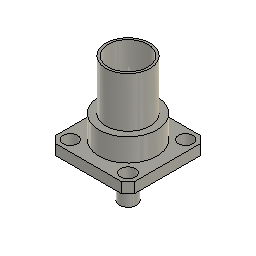
sBitx V3 radio aj6cu v1 (Autodesk Fusion 360 archive; units mm, degrees)
design "BNC connector"
Autodesk Fusion 360 part; units mm, degrees
sketch "Sketch1" plane through (0, 0, 0) normal (0, 1, 0) x (1, 0, 0) in component "BNC 4-hole panel mount"
  line L0 (-6.35, -9.3) -> (-8.75, -9.3)
  line L1 (-8.75, -9.3) -> (-8.75, -11.6)
  line L2 (-8.75, -11.6) -> (-6.35, -11.6)
  line L3 (-6.35, -11.6) -> (-6.35, -16.6)
  line L4 (-6.35, -16.6) -> (-4.85, -16.6)
  line L5 (-4.85, -16.6) -> (-4.85, -27.6)
  line L6 (0, -27.6) -> (0, 0)
  line L7 (-6.35, -9.3) -> (-6.35, -7.3)
  line L8 (-6.35, -7.3) -> (-1.9, -7.3)
  line L9 (-1.9, -7.3) -> (-1.9, 0)
  line L10 (0, 0) -> (-1.9, 0)
  line L11 (-4.85, -27.6) -> (-4.35, -27.6)
  line L12 (-4.35, -27.6) -> (-4.35, -14.6)
  line L13 (-4.35, -14.6) -> (-0.6, -14.6)
  line L14 (-0.6, -14.6) -> (-0.6, -24.1)
  line L15 (-0.6, -24.1) -> (0, -25.6)
  dimension "d3" = 1.9
  dimension "d4" = 2.3
  dimension "d5" = 5
  dimension "d6" = 8.75
  dimension "d9" = 4.85
  dimension "d10" = 6.35
  dimension "d11" = 2
  dimension "d21" = 0.5
  dimension "d22" = 0.6
  dimension "d23" = 1.5
  dimension "d24" = 13
  dimension "d25" = 27.6
  dimension "d26" = 11
  dimension "d27" = 16
  constraint perpendicular L0 L1
  constraint perpendicular L1 L2
  constraint perpendicular L2 L3
  constraint perpendicular L3 L4
  constraint perpendicular L4 L5
  constraint vertical L6
  constraint coincident L6.end L10.start
  constraint perpendicular L0 L7
  constraint perpendicular L7 L8
  constraint perpendicular L8 L9
  constraint perpendicular L9 L10
  constraint collinear L3 L7
  constraint perpendicular L5 L11
  constraint perpendicular L11 L12
  constraint perpendicular L12 L13
  constraint perpendicular L13 L14
  constraint coincident L6 L15.end
  measures "d3" distance of L6 L9
  measures "d4" distance of L0.end L1.end
  measures "d5" distance of L2 L4
  measures "d6" distance of L1 L6
  measures "d9" distance of L5 L6
  measures "d10" distance of L3 L6
  measures "d11" distance of L0 L8
  measures "d21" distance of L5 L12
  measures "d22" distance of L6 L14
  measures "d23" vertical distance of L14.end L15.end
  measures "d24" distance of L11.end L12.end
  measures "d25" vertical distance of L6.end L5.end
  measures "d26" distance of L13 L15.end
  measures "d27" distance of L2 L5.end
revolve "Revolve1" add sketch "Sketch1" angle 360 about axis through (0, 0, 27.6) along (0, 0, -1) in component "BNC 4-hole panel mount"
sketch "Sketch2" plane through (0, 0, 11.6) normal (0, 0, 1) x (-1, 0, 0) in component "BNC 4-hole panel mount"
  circle A0 centre (0, 0) radius 6.35
  circle A1 centre (0, 0) radius 8.75
  line L0 (8.75, -8.75) -> (-8.75, -8.75)
  line L1 (-8.75, -8.75) -> (-8.75, 8.75)
  line L2 (-8.75, 8.75) -> (8.75, 8.75)
  line L3 (8.75, 8.75) -> (8.75, -8.75)
  line L4 (8.75, -8.75) -> (-8.75, 8.75) construction
  line L5 (-8.75, -8.75) -> (8.75, 8.75) construction
  circle A2 centre (6.35, 6.35) radius 1.6
  circle A3 centre (6.35, -6.35) radius 1.6
  circle A4 centre (-6.35, -6.35) radius 1.6
  circle A5 centre (-6.35, 6.35) radius 1.6
  circle A6 centre (0, 0) radius 6.35
  dimension "d13" = 17.5
  dimension "d14" = 17.5
  dimension "d15" = 3.2
  dimension "d16" = 12.7
  constraint horizontal L0
  constraint perpendicular L0 L1
  constraint parallel L0 L2
  constraint parallel L1 L3
  constraint coincident L4 A0.centre
  constraint coincident L5 A0.centre
  constraint coincident A0.centre A1.centre
  constraint coincident L5 A2.centre
  constraint coincident L4 A3.centre
  constraint coincident L5 A4.centre
  constraint coincident L4 A5.centre
  constraint equal A4 A5
  constraint equal A3 A4
  constraint equal A2 A5
  constraint horizontal A2.centre A5.centre
  constraint horizontal A3.centre A4.centre
  constraint vertical A4.centre A5.centre
  measures "d13" distance of L1.end L2.end
  measures "d14" distance of L0.end L1.end
  measures "d15" diameter of A5
  measures "d16" horizontal distance of A2.centre A5.centre
extrude "Extrude1" add sketch "Sketch2" against normal up to surface (2.3 mm away) contours A1 A2 A3 A4 A5 | A1 L0 L3 A3 | A1 L2 L3 A2 | A1 L1 L2 A5 | A1 L0 L1 A4 in component "BNC 4-hole panel mount"
extrude "Extrude2" cut sketch "Sketch2" against normal up to surface (2.3 mm away) contours A1 A2 | A1 A3 | A1 A5 | A1 A4 picked at (5.857, 5.857) picked at (5.857, -5.857) picked at (-5.8818, 5.8337) picked at (-5.8818, -5.8337) in component "BNC 4-hole panel mount"
chamfer "Chamfer1" distance 1.5 angle 45 4 edges at (8.75, -8.75, 10.45) (-8.75, -8.75, 10.45) (-8.75, 8.75, 10.45) (8.75, 8.75, 10.45) in component "BNC 4-hole panel mount"
component "BNC 4-hole panel mount" placed x (1, 0, 0) y (0, 1, 0) z (0, 0, 1) at (0, 0, 0)
equation "d14 = d13"
